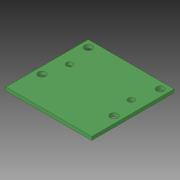
# Autodesk Inventor part: Waveshare Kamera PCB 24x25
Saved by Autodesk Inventor 2019.1 (Build 231200000, 200)
## iProperties
Part Number: Waveshare Kamera PCB 24x25
Material: Phenolharz
Document SubType Name: Modeling
Designer: rYan
Mass: 0.799836 g
Surface Area: 12.9626 cm^2
Volume: 0.579592 cm^3
Density: 1.38 g/cm^3
Appearance: Glatt - waldgrün
Author: rYan
Autodesk Inventor part; units mm, degrees
ref_plane "YZ Plane" through (0, 0, 0) normal (1, 0, 0) x (0, 1, 0)
ref_plane "XZ Plane" through (0, 0, 0) normal (0, 1, 0) x (-1, 0, 0)
ref_plane "XY Plane" through (0, 0, 0) normal (0, 0, 1) x (1, 0, 0)
sketch "Skizze1" plane through (0, 0, 0) normal (0, 0, 1) x (1, 0, 0)
  line L0 (-12.5, -12) -> (12.5, -12)
  line L1 (12.5, -12) -> (12.5, 12)
  line L2 (12.5, 12) -> (-12.5, 12)
  line L3 (-12.5, 12) -> (-12.5, -12)
  line L4 (-12.5, -12) -> (12.5, 12) construction
  line L5 (12.5, -12) -> (-12.5, 12) construction
  point P0 (0, 0)
  dimension "d0" = 25
  dimension "d1" = 24
  constraints: 12 end point, 2 midpoint, 2 parallel, 1 horizontal, 1 perpendicular
  measures "d0" distance of L2.end L1.end
  measures "d1" distance of L1.end L0.end
extrude "Extrusion1" add sketch "Skizze1" along normal blind 1
sketch "Skizze2" plane through (0, 0, 1) normal (0, 0, 1) x (1, 0, 0)
  line L0 (-12.5, -12) -> (12.5, -12) projected
  line L1 (12.5, -12) -> (12.5, 12) projected
  line L2 (12.5, 12) -> (-12.5, 12) projected
  line L3 (-12.5, 12) -> (-12.5, -12) projected
  line L4 (12.5, 12) -> (-12.5, 12) construction
  line L5 (0, 12) -> (0, -12) construction
  line L6 (-12.5, -12) -> (12.5, -12) construction
  point P0 (0, 0)
  point P1 (-10.5, 10)
  point P2 (10.5, 10)
  point P3 (10.5, -3.5)
  point P4 (-10.5, -3.5)
  dimension "d4" = 2
  dimension "d5" = 2
  dimension "d6" = 8.5
  dimension "d7" = 2
  constraints: 2 end point, 2 midpoint, 2 symmetric about line
  measures "d4" distance from line of L2 point (-10.5, 10)
  measures "d5" distance from line of L3 point (-10.5, 10)
  measures "d6" distance from line of L0 point (-10.5, -3.5)
  measures "d7" distance from line of L3 point (-10.5, -3.5)
hole "Bohrung1" at (-10.5, 10, 1) at (10.5, 10, 1) at (10.5, -3.5, 1) at (-10.5, -3.5, 1) direction (0, 0, -1) diameter 2.2 end through all
sketch "Skizze3" plane through (0, 0, 1) normal (0, 0, 1) x (1, 0, 0)
  circle A0 centre (10.5, -3.5) radius 1.1 projected
  circle A1 centre (-10.5, 10) radius 1.1 projected
  circle A2 centre (10.5, 10) radius 1.1 projected
  circle A3 centre (-10.5, -3.5) radius 1.1 projected
  line L0 (-12.5, -12) -> (12.5, -12) projected
  line L1 (12.5, -12) -> (12.5, 12) projected
  line L2 (12.5, 12) -> (-12.5, 12) projected
  line L3 (-12.5, 12) -> (-12.5, -12) projected
  line L4 (0, 12) -> (0, -12) construction
  point P0 (0, 0)
  point P1 (-9, 3)
  point P2 (9, 3)
  dimension "d16" = 9
  dimension "d17" = 18
  constraints: 2 end point, 2 midpoint, 1 symmetric about line
  measures "d16" distance from line of L2 point (-9, 3)
  measures "d17" distance of point (9, 3) point (-9, 3)
hole "Bohrung2" at (-9, 3, 1) at (9, 3, 1) direction (0, 0, -1) diameter 1.82 end through all
